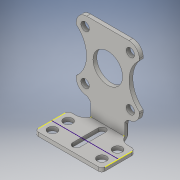
# Autodesk Inventor part: motor mount sumo Jeffrey P
Saved by Autodesk Inventor 2016 (Build 200138000, 138)
## iProperties
Created: 2017-09-05
Part Number: motor mount sumo Jeffrey P
Material: Generic
Document SubType Name: Modeling
Designer: student
Density: 1 g/cm^3
Appearance: Default
Author: student
Autodesk Inventor part; units mm, degrees
ref_plane "YZ Plane" through (0, 0, 0) normal (1, 0, 0) x (0, 1, 0)
ref_plane "XZ Plane" through (0, 0, 0) normal (0, 1, 0) x (-1, 0, 0)
ref_plane "XY Plane" through (0, 0, 0) normal (0, 0, 1) x (1, 0, 0)
sketch "Sketch1" plane through (0, 0, 0) normal (0, 0, 1) x (1, 0, 0)
  line L0 (-6.985, -11.3792) -> (6.985, -11.3792)
  line L1 (6.985, 11.3792) -> (-6.985, 11.3792)
  line L2 (-10.414, -11.3792) -> (10.414, 11.3792) construction
  line L3 (10.414, -11.3792) -> (-10.414, 11.3792) construction
  circle A0 centre (0, 0) radius 4.9022
  line L4 (10.414, 11.3792) -> (-10.414, -11.3792) construction
  arc A1 (-6.985, 11.3792) -> (-10.414, 7.9502) centre (-6.985, 7.9502) ccw
  arc A2 (10.414, 7.9502) -> (6.985, 11.3792) centre (6.985, 7.9502) ccw
  arc A3 (6.985, -11.3792) -> (10.414, -7.9502) centre (6.985, -7.9502) ccw
  arc A4 (-10.414, -7.9502) -> (-6.985, -11.3792) centre (-6.985, -7.9502) ccw
  circle A5 centre (-7.48241, 8.175901) radius 1.397
  circle A6 centre (7.48241, 8.175901) radius 1.397
  circle A7 centre (-7.48241, -8.175901) radius 1.397
  circle A8 centre (7.48241, -8.175901) radius 1.397
  arc A9 (-10.414, -7.321195) -> (-10.414, 7.321195) centre (-16.5862, 0) ccw
  arc A10 (10.414, 7.321195) -> (10.414, -7.321195) centre (16.5862, 0) ccw
  line L5 (-10.414, -7.9502) -> (-10.414, -7.321195)
  line L6 (-10.414, 7.321195) -> (-10.414, 7.9502)
  line L7 (10.414, -7.9502) -> (10.414, -7.321195)
  line L8 (10.414, 7.321195) -> (10.414, 7.9502)
  dimension "d0" = 22.7584
  dimension "d1" = 20.828
  dimension "d2" = 9.8044
  dimension "d9" = 3.429
  dimension "d10" = 2.794
  dimension "d18" = 2.1082
  dimension "d20" = 9.5758
  constraints: 18 end point, 12 point on circle, 12 tangent, 11 centre point, 5 point on line, 3 equal radius, 2 midpoint, 2 perpendicular, 2 vertical, 1 coincident, 1 horizontal, 1 parallel
  measures "d0" distance of L3.start L2.end
  measures "d1" distance of L2.end L3.end
  measures "d2" diameter of A0
  measures "d9" radius of A1
  measures "d10" diameter of A5
  measures "d20" radius of A10
extrude "Extrusion1" add sketch "Sketch1" along normal blind 1.27
sketch "Sketch3" plane through (0, 0, 0) normal (0, 0, -1) x (-1, 0, 0)
  line L0 (-5.407328, -16.764) -> (5.407328, -16.764)
  line L1 (5.407328, -16.764) -> (5.407328, -13.797073)
  line L2 (-5.407328, -13.797073) -> (-5.407328, -16.764)
  line L3 (6.985, -11.3792) -> (-6.985, -11.3792)
  line L4 (-5.407328, -16.764) -> (3.619749, -7.774531) construction
  line L5 (5.407328, -16.764) -> (-3.619749, -7.774531) construction
  line L6 (-5.407328, -11.3792) -> (5.407328, -11.3792)
  arc A0 (-5.407328, -13.797073) -> (-6.985, -11.3792) centre (-8.048928, -13.797073) ccw
  arc A1 (6.985, -11.3792) -> (5.407328, -13.797073) centre (8.048928, -13.797073) ccw
  point P0 (0, 0)
  point P1 (0, -11.3792)
  dimension "d28" = 5.3848
  dimension "d29" = 2.6416
  constraints: 12 end point, 6 point on line, 4 point on circle, 2 centre point, 2 perpendicular, 2 tangent, 1 equal radius, 1 horizontal, 1 midpoint, 1 parallel
  measures "d28" distance of L0.end L6.end
  measures "d29" radius of A0
extrude "Extrusion3" add sketch "Sketch3" against normal blind 1.27
sketch "Sketch4" plane through (-5.407328, -16.764, 0) normal (0, -1, 0) x (1, 0, 0)
  point P0 (5.407328, 0)
sketch "Sketch5" plane through (0, 0, 1.27) normal (0, 0, 1) x (1, 0, 0)
  point P0 (5.407328, -16.764)
  point P1 (-5.407328, -16.764)
sketch "Sketch6" plane through (-5.407328, -16.764, 0) normal (0, -1, 0) x (1, 0, 0)
  line L0 (0, 1.27) -> (10.814656, 1.27)
  line L1 (0, 1.27) -> (10.814656, 1.27)
  line L2 (10.814656, 1.27) -> (10.814656, 3.302)
  line L3 (10.814656, 3.302) -> (0, 3.302)
  line L4 (0, 3.302) -> (0, 1.27)
  dimension "d57" = 2.032
  constraints: 8 end point, 3 equal length, 1 perpendicular
  measures "d57" distance of L0.end L2.end
sketch "Sketch7" plane through (-5.407328, -16.764, 0) normal (0, -1, 0) x (1, 0, 0)
  line L0 (10.814656, 0) -> (10.814656, 1.27)
  line L1 (0, 0) -> (0, 1.27)
  line L2 (10.814656, 0) -> (0, 0)
  line L3 (0, 0) -> (0, 1.27)
  line L4 (0, 1.27) -> (10.814656, 1.27)
  line L5 (10.814656, 1.27) -> (10.814656, 0)
  point P0 (5.407328, 0)
  constraints: 8 end point, 2 parallel, 1 horizontal, 1 perpendicular
extrude "Extrusion5" add sketch "Sketch7" along normal blind 1.27
fillet "Fillet1" radius 1.27 1 edges at (0, -18.034, 0)
extrude "Extrusion8" add sketch "Sketch6" along normal blind 1.27
sketch "Sketch10" plane through (-5.407328, -16.764, 0) normal (0, 1, 0) x (1, 0, 0)
  line L0 (10.814656, -1.27) -> (10.814656, -3.302)
  line L1 (-5.616272, -3.302) -> (16.430928, -3.302)
  line L2 (16.430928, -3.302) -> (16.430928, -14.3002)
  line L3 (16.430928, -14.3002) -> (-5.616272, -14.3002)
  line L4 (-5.616272, -14.3002) -> (-5.616272, -3.302)
  line L5 (10.814656, -3.302) -> (0, -3.302)
  point P0 (5.407328, 0)
  point P1 (5.407328, -3.302)
  dimension "d61" = 22.0472
  dimension "d62" = 10.9982
  constraints: 8 end point, 2 midpoint, 2 parallel, 1 collinear, 1 perpendicular
  measures "d61" distance between parallel lines of L2 L4
  measures "d62" distance of L1.end L2.end
extrude "Extrusion9" add sketch "Sketch10" against normal blind 1.27
fillet "Fillet2" radius 3.175 2 edges at (5.4073, -17.399, 3.302) (-5.4073, -17.399, 3.302)
sketch "Sketch11" plane through (-5.407328, -16.764, 0) normal (0, 1, 0) x (1, 0, 0)
  point P0 (5.407328, 0)
fillet "Fillet3" radius 1.016 4 edges at (-11.0236, -17.399, 3.302) (-11.0236, -17.399, 14.3002) (11.0236, -17.399, 14.3002) (11.0236, -17.399, 3.302)
sketch "Sketch12" plane through (-5.407328, -16.764, 0) normal (0, 1, 0) x (1, 0, 0)
  line L0 (-5.616272, -13.2842) -> (-5.616272, -4.318)
  line L1 (16.430928, -4.318) -> (16.430928, -13.2842)
  line L2 (15.414928, -14.3002) -> (-4.600272, -14.3002)
  line L3 (-0.212876, -1.27) -> (11.027532, -1.27)
  circle A0 centre (-2.758772, -6.2103) radius 1.5113
  line L4 (-4.600272, -3.302) -> (-3.175, -3.302)
  arc A1 (-3.175, -3.302) -> (-0.212876, -1.27) centre (-3.175, -0.127) ccw
  line L5 (-5.616272, -8.8011) -> (16.430928, -8.8011)
  circle A2 centre (-2.758772, -11.3919) radius 1.5113
  line L6 (15.414928, -14.3002) -> (-4.600272, -14.3002)
  line L7 (5.407328, -14.3002) -> (5.407328, -1.27)
  line L8 (10.309528, -1.27) -> (0.505128, -1.27)
  circle A3 centre (13.573428, -6.2103) radius 1.5113
  circle A4 centre (13.573428, -11.3919) radius 1.5113
  line L9 (5.407328, -3.2258) -> (5.407328, -11.6586) construction
  line L10 (4.162728, -3.2258) -> (4.162728, -11.6586)
  line L11 (6.651928, -11.6586) -> (6.651928, -3.2258)
  arc A5 (6.651928, -3.2258) -> (4.162728, -3.2258) centre (5.407328, -3.2258) ccw
  arc A6 (4.162728, -11.6586) -> (6.651928, -11.6586) centre (5.407328, -11.6586) ccw
  point P0 (5.407328, 0)
  point P1 (5.407328, -7.4422)
  dimension "d69" = 3.0226
  dimension "d74" = 2.6416
  dimension "d75" = 1.9558
  dimension "d76" = 2.4892
  dimension "d79" = 2.159
  dimension "d80" = 13.3096
  dimension "d81" = 2.9083
  dimension "d82" = 2.8575
  constraints: 12 end point, 6 centre point, 5 midpoint, 4 point on circle, 4 tangent, 3 symmetric about line, 2 point on line, 1 parallel, 3 other
  measures "d69" diameter of A0
  measures "d74" distance from line of L2 L9.end
  measures "d75" distance from line of L8 L9.start
  measures "d76" distance between parallel lines of L11 L10
  measures "d81" distance from line of L6 A4.centre
  measures "d82" distance from line of L0 A2.centre
sketch "Sketch13" plane through (-5.407328, -16.764, 0) normal (0, 1, 0) x (1, 0, 0)
  line L0 (-5.616272, -13.2842) -> (-5.616272, -4.318)
  line L1 (-5.616272, -8.8011) -> (16.430928, -8.8011)
  line L2 (16.430928, -4.318) -> (16.430928, -13.2842)
  point P0 (5.407328, 0)
  constraints: 2 end point, 2 midpoint
extrude "Extrusion10" cut sketch "Sketch12" against normal blind 1.27
sketch "Sketch14" plane through (-5.407328, -16.764, 0) normal (0, 1, 0) x (1, 0, 0)
  point P0 (5.407328, 0)
body "Solid1"
